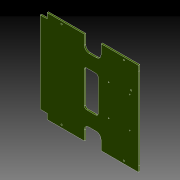
# Autodesk Inventor part: KB33-046-004-018 - Полка электроники
Saved by Autodesk Inventor 2020 (Build 240168000, 168)
## iProperties
Created: 2021-06-26
Part Number: KB33-046-004-018 - Полка электроники
Material: Типовые
Document SubType Name: Modeling
Designer: Петров Иван
Mass: 244.165 g
Surface Area: 1282.82 cm^2
Volume: 244.165 cm^3
Density: 1 g/cm^3
Appearance: По умолчанию
Author: Петров Иван
Autodesk Inventor part; units mm, degrees
ref_plane "YZ Plane" through (0, 0, 0) normal (1, 0, 0) x (0, 1, 0)
ref_plane "XZ Plane" through (0, 0, 0) normal (0, 1, 0) x (-1, 0, 0)
ref_plane "XY Plane" through (0, 0, 0) normal (0, 0, 1) x (1, 0, 0)
sketch "Эскиз1" plane through (0, 0, 0) normal (0, 0, 1) x (1, 0, 0)
  circle A0 centre (25, 157.5) radius 2
  circle A1 centre (196.5682, 157.5) radius 2
  line L0 (236.5682, 150) -> (236.5682, 165) projected
  line L1 (-34.0192, 150) -> (-15, 150)
  line L2 (-34.0192, 150) -> (-15, 150)
  line L3 (-34.0192, 37.5) -> (-34.0192, 150)
  line L4 (236.5682, 165) -> (-15, 165)
  line L5 (236.5682, 37.5) -> (236.5682, 165)
  line L6 (-34.0192, 37.5) -> (236.5682, 37.5)
  line L7 (-15, 165) -> (-15, 150)
  dimension "d5" = 127.5
  dimension "d6" = 7.5
  dimension "d7" = 7.5
  dimension "d9" = 15
  constraints: 14 end point, 2 centre point, 1 horizontal, 1 vertical
  measures "d5" distance between parallel lines of L6 L4
  measures "d6" distance from line of L4 A1.centre
  measures "d7" distance from line of L4 A0.centre
  measures "d9" distance of L4.end L1.end
extrude "Выдавливание1" add sketch "Эскиз1" along normal blind 4
sketch "Эскиз2" plane through (0, 0, 4) normal (0, 0, 1) x (1, 0, 0)
  line L0 (236.5682, 150) -> (199.2972, 150)
  line L1 (-15, 150) -> (-34.0192, 150) projected
  line L2 (-34.0192, 37.5) -> (236.5682, 37.5) projected
  line L3 (199.2972, 150) -> (236.5682, 150)
  line L4 (236.5682, 150) -> (236.5682, 37.5)
  line L5 (236.5682, 37.5) -> (199.2972, 37.5)
  line L6 (199.2972, 37.5) -> (199.2972, 150)
  point P0 (0, 0)
  point P1 (-24.5096, 150)
  point P2 (-15, -15)
  constraints: 10 end point, 2 horizontal, 2 parallel, 1 horizontal alignment, 1 midpoint, 1 perpendicular
extrude "Выдавливание2" cut sketch "Эскиз2" against normal blind 4
mirror "Зеркальное отражение2" about plane through (-34.0192, 37.5, 0) normal (0, -1, 0) of "Выдавливание1", "Выдавливание2"
sketch "Эскиз3" plane through (0, 0, 4) normal (0, 0, 1) x (1, 0, 0)
  line L0 (236.5682, -90) -> (-15, -90) projected
  line L1 (87.4676, -90) -> (133.662, -90)
  line L2 (133.662, -90) -> (133.662, -50.4003)
  line L3 (133.662, -50.4003) -> (87.4676, -50.4003)
  line L4 (87.4676, -50.4003) -> (87.4676, -90)
  point P0 (0, 0)
  constraints: 8 end point, 2 parallel, 1 horizontal, 1 perpendicular, 1 point on line
extrude "Выдавливание3" cut sketch "Эскиз3" against normal blind 10
ref_plane "РабПлоскость1" through (199.2972, 37.5, 4) normal (0, 1, 0) x (1, 0, 0)
mirror "Зеркальное отражение3" about plane through (199.2972, 37.5, 4) normal (0, 1, 0) of "Выдавливание3"
move faces "Перенос1" translate (37.25, 0, 0) faces at (199.2972, 0, 2.6667)
sketch "Эскиз4" plane through (0, 0, 4) normal (0, 0, 1) x (1, 0, 0)
  circle A0 centre (154.5472, 83.5) radius 1.375 projected
  circle A1 centre (154.5472, -2.5) radius 1.375 projected
  circle A2 centre (212.5472, -2.5) radius 1.375 projected
  circle A3 centre (212.5472, 83.5) radius 1.375 projected
  circle A4 centre (216.5472, 95.5) radius 2 projected
  circle A5 centre (216.5472, -20.5) radius 2 projected
  line L0 (215.9472, 87.5) -> (138.1472, 87.5) projected
  line L1 (138.1472, -12.5) -> (215.9472, -12.5) projected
  line L2 (125.662, 87.5) -> (87.4676, 87.5)
  line L3 (87.4676, 87.5) -> (87.4676, -12.5)
  line L4 (87.4676, -12.5) -> (125.662, -12.5)
  line L5 (125.662, -12.5) -> (125.662, 87.5)
  line L6 (87.4676, -90) -> (87.4676, -50.4003) projected
  line L7 (133.662, -50.4003) -> (133.662, -90) projected
  point P0 (0, 0)
  dimension "d15" = 8
  constraints: 8 end point, 2 parallel, 1 horizontal, 1 perpendicular, 1 point on line
  measures "d15" distance between parallel lines of L7 L5
extrude "Выдавливание4" cut sketch "Эскиз4" against normal blind 10 contours A0 | A1 | A2 | A3 | A4 | L5 L4 L3 L2
fillet "Сопряжение1" radius 13 4 edges at (87.4676, 125.4003, 2) (133.662, 125.4003, 2) (87.4676, -50.4003, 2) (133.662, -50.4003, 2)
fillet "Сопряжение2" radius 6.5 4 edges at (87.4676, -12.5, 2) (125.662, -12.5, 2) (87.4676, 87.5, 2) (125.662, 87.5, 2)
